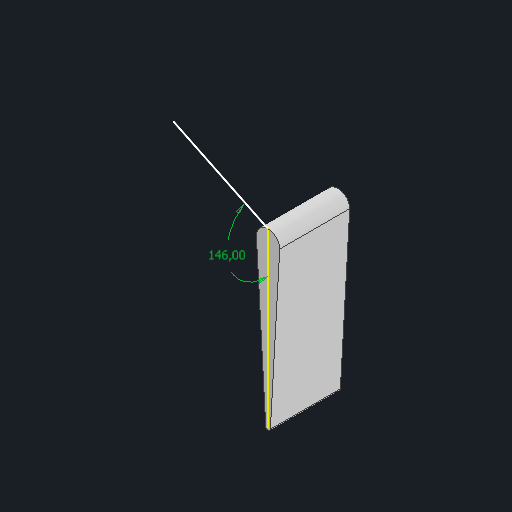
# Autodesk Inventor part: дворник 25-26
Saved by Autodesk Inventor 2025 (Build 290162000, 162)
## iProperties
Created: 2025-10-08
Part Number: дворник 25-26
Material: Типовые
Document SubType Name: Modeling
Designer: Phantom
Density: 1 g/cm^3
Appearance: По умолчанию
Author: Phantom
Autodesk Inventor part; units mm, degrees
ref_plane "YZ Plane" through (0, 0, 0) normal (1, 0, 0) x (0, 1, 0)
ref_plane "XZ Plane" through (0, 0, 0) normal (0, 1, 0) x (-1, 0, 0)
ref_plane "XY Plane" through (0, 0, 0) normal (0, 0, 1) x (1, 0, 0)
sketch "Эскиз1" plane through (0, 0, 0) normal (0, 0, 1) x (1, 0, 0)
  circle A0 centre (0, 0) radius 5
  line L0 (0, 0) -> (0, -86)
  line L1 (0, -86) -> (-5, 0)
  line L2 (0, -86) -> (5, 0)
  dimension "d0" = 10
  dimension "d1" = 86
  constraints: 6 end point, 2 point on circle, 1 centre point, 1 coincident, 1 vertical
  measures "d0" diameter of A0
  measures "d1" distance of L0.start L0.end
extrude "Выдавливание1" add sketch "Эскиз1" along normal blind 30 contours L2 A0 L1 | L2 L0 A0 | A0 L0 L1
fillet "Сопряжение1" radius 1 1 edges at (0, -86, 15)
sketch "Эскиз2" plane through (0, 0, 0) normal (1, 0, 0) x (0, 1, 0)
  line L0 (-68.829, 30) -> (0, 30) projected
  line L1 (5, 30) -> (0, 30) projected
  line L2 (5, 30) -> (64.7655, 70.3123)
  point P0 (0, 0)
  dimension "d5" = 146
  constraints: 2 end point
  measures "d5" angle of L2 L0
